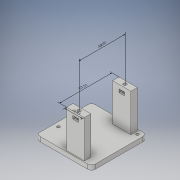
# Autodesk Inventor part: MotorHolder
Saved by Autodesk Inventor 2019 (Build 230136000, 136)
## iProperties
Created: 2018-06-26
Part Number: MotorHolder
Material: Ogólny
Document SubType Name: Modeling
Designer: Kamil
Density: 1 g/cm^3
Appearance: Domyślna
Author: Kamil
## iProperties of the stored document MotorHolder_Drukowanie 3D.ipt
Created: 2018-06-26
Part Number: MotorHolder_Drukowanie 3D
Material: Ogólny
Document SubType Name: Modeling
Designer: Kamil
Density: 1 g/cm^3
Appearance: Domyślna
Author: Kamil
Autodesk Inventor part; units mm, degrees
ref_plane "YZ Plane" through (0, 0, 0) normal (1, 0, 0) x (0, 1, 0)
ref_plane "XZ Plane" through (0, 0, 0) normal (0, 1, 0) x (-1, 0, 0)
ref_plane "XY Plane" through (0, 0, 0) normal (0, 0, 1) x (1, 0, 0)
sketch "Szkic1" plane through (0, 0, 0) normal (0, 1, 0) x (-1, 0, 0)
  line L0 (-26, 30) -> (26, 30)
  line L1 (30, 26) -> (30, -26)
  line L2 (26, -30) -> (-26, -30)
  line L3 (-30, -26) -> (-30, 26)
  line L4 (-30, 30) -> (30, -30) construction
  line L5 (30, 30) -> (-30, -30) construction
  circle A0 centre (-25, -25) radius 1.5
  circle A1 centre (25, 11) radius 1.5
  arc A2 (-30, -26) -> (-26, -30) centre (-26, -26) ccw
  arc A3 (-26, 30) -> (-30, 26) centre (-26, 26) ccw
  arc A4 (30, 26) -> (26, 30) centre (26, 26) ccw
  arc A5 (26, -30) -> (30, -26) centre (26, -26) ccw
  point P0 (0, 0)
  dimension "d0" = 60
  dimension "d1" = 60
  dimension "d2" = 3
  dimension "d3" = 3
  dimension "d5" = 4
  dimension "d6" = 4
  dimension "d7" = 4
  dimension "d8" = 4
  constraints: 12 end point, 8 point on circle, 8 point on line, 8 tangent, 6 centre point, 2 midpoint, 2 parallel, 1 horizontal, 1 perpendicular
  measures "d0" distance of L4.end L5.end
  measures "d1" distance of L5.start L4.end
  measures "d2" diameter of A0
  measures "d3" diameter of A1
  measures "d5" radius of A2
  measures "d6" radius of A3
  measures "d7" radius of A4
  measures "d8" radius of A5
extrude "Wyciągnięcie proste1" add sketch "Szkic1" along normal blind 5
sketch "Szkic2" plane through (0, 5, 0) normal (0, 1, 0) x (1, 0, 0)
  line L0 (21.8475, 21.1097) -> (1.8475, 21.1097)
  line L1 (1.8475, 21.1097) -> (1.8475, 28.1097)
  line L2 (1.8475, 28.1097) -> (21.8475, 28.1097)
  line L3 (21.8475, 28.1097) -> (21.8475, 21.1097)
  line L4 (1.8475, -22) -> (21.2771, -22)
  line L5 (21.2771, -22) -> (21.2771, -29)
  line L6 (21.2771, -29) -> (1.8475, -29)
  line L7 (1.8475, -29) -> (1.8475, -22)
  point P0 (0, 0)
  dimension "d11" = 20
  dimension "d12" = 7
  dimension "d13" = 7
  constraints: 16 end point, 4 parallel, 2 horizontal, 2 perpendicular, 1 point on line
  measures "d11" distance of L1.end L2.end
  measures "d12" distance of L0.end L1.end
  measures "d13" distance of L4.end L5.end
extrude "Wyciągnięcie proste2" add sketch "Szkic2" along normal blind 41
sketch "Szkic3" plane through (1.8475, 5, 29) normal (0, 0, 1) x (1, 0, 0)
  line L0 (7, 33.2857) -> (13, 33.2857)
  line L1 (13, 33.2857) -> (13, 36.7143)
  line L2 (13, 36.7143) -> (7, 36.7143)
  line L3 (7, 36.7143) -> (7, 33.2857)
  line L4 (7, 33.2857) -> (13, 36.7143) construction
  line L5 (13, 33.2857) -> (7, 36.7143) construction
  point P0 (-1.8475, -5)
  point P1 (10, 35)
  dimension "d16" = 6
  dimension "d17" = 3.4286
  constraints: 12 end point, 2 midpoint, 2 parallel, 1 horizontal, 1 perpendicular
  measures "d16" distance of L2.end L1.end
  measures "d17" distance of L1.end L0.end
sketch "Szkic4" plane through (1.8475, 5, -21.1097) normal (0, 0, 1) x (1, 0, 0)
  line L0 (7, 33.2857) -> (13, 33.2857)
  line L1 (13, 33.2857) -> (13, 36.7143)
  line L2 (13, 36.7143) -> (7, 36.7143)
  line L3 (7, 36.7143) -> (7, 33.2857)
  line L4 (7, 33.2857) -> (13, 36.7143) construction
  line L5 (13, 33.2857) -> (7, 36.7143) construction
  point P0 (-1.8475, -5)
  point P1 (10, 35)
  dimension "d18" = 6
  dimension "d19" = 3.4286
  constraints: 12 end point, 2 midpoint, 2 parallel, 1 horizontal, 1 perpendicular
  measures "d18" distance of L3.start L4.end
  measures "d19" distance of L4.end L1.start
extrude "Wyciągnięcie proste3" cut sketch "Szkic4" against normal blind 7
extrude "Wyciągnięcie proste4" cut sketch "Szkic3" against normal blind 7
sketch "Szkic5" plane through (0, 46, 0) normal (0, 1, 0) x (1, 0, 0)
  circle A0 centre (12, 24.5) radius 1.75
  circle A1 centre (12, -25.5) radius 1.75
  point P0 (0, 0)
  dimension "d24" = 3.5
  dimension "d25" = 3.5
  constraints: 2 centre point
  measures "d24" diameter of A0
  measures "d25" diameter of A1
extrude "Wyciągnięcie proste5" cut sketch "Szkic5" against normal blind 20
